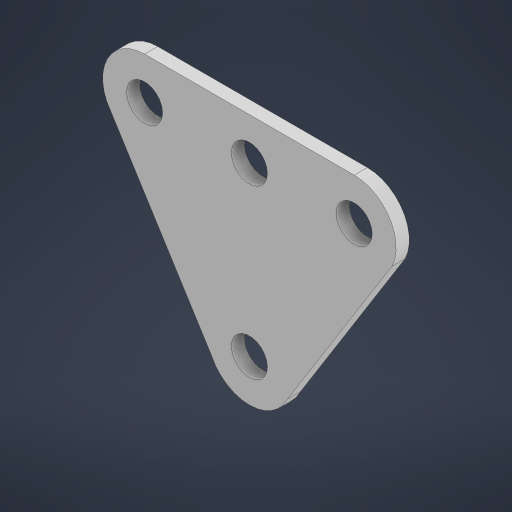
# Autodesk Inventor part: Wing poly connection
Saved by Autodesk Inventor 2023.4 (Build 274418000, 418)
## iProperties
Created: 2024-01-13
Part Number: Wing poly connection
Material: Generic
Document SubType Name: Modeling
Designer: diego
Density: 1 g/cm^3
Appearance: Default
Author: diego
Autodesk Inventor part; units mm, degrees
ref_plane "YZ Plane" through (0, 0, 0) normal (1, 0, 0) x (0, 1, 0)
ref_plane "XZ Plane" through (0, 0, 0) normal (0, 1, 0) x (-1, 0, 0)
ref_plane "XY Plane" through (0, 0, 0) normal (0, 0, 1) x (1, 0, 0)
sketch "Sketch3" plane through (0, 0, 0) normal (0, 0, 1) x (1, 0, 0)
  circle A0 centre (1.4019, 6.1779) radius 2.1844
  circle A1 centre (-11.2981, 6.1779) radius 2.1844
  circle A2 centre (-23.9981, 6.1779) radius 2.1844
  circle A3 centre (14.1019, 6.1779) radius 2.1844
  line L0 (-11.2981, 6.1779) -> (1.4019, 6.1779)
  line L1 (1.4019, 6.1779) -> (14.1019, 6.1779)
  circle A4 centre (-11.2981, 6.1779) radius 5.08
  circle A5 centre (1.4019, 6.1779) radius 5.08
  circle A6 centre (14.1019, 6.1779) radius 5.08
  line L2 (-11.2981, 11.2579) -> (1.4019, 11.2579)
  line L3 (1.4019, 11.2579) -> (14.1019, 11.2579)
  line L4 (1.4019, 6.1779) -> (1.4019, -14.1421)
  circle A7 centre (1.4019, -14.1421) radius 5.08
  circle A8 centre (1.4019, -14.1421) radius 2.1844
  line L5 (-15.8845, 3.9935) -> (-3.1845, -16.3265)
  line L6 (5.9882, -16.3265) -> (18.6882, 3.9935)
  point P0 (0, 0)
  dimension "d55" = 10.16
  dimension "d54" = 10.16
  dimension "d56" = 10.16
  dimension "d57" = 20.32
  dimension "d58" = 10.16
  dimension "d59" = 4.3688
  dimension "d60" = 4.3688
  constraints: 14 end point, 8 centre point, 6 point on circle, 5 coincident, 2 horizontal, 1 collinear, 1 point on line, 1 vertical, 1 vertical alignment, 2 other
  measures "d54" diameter of A4
  measures "d56" diameter of A6
  measures "d57" distance of L4.start L4.end
  measures "d58" diameter of A7
  measures "d59" diameter of A3
  measures "d60" diameter of A8
extrude "Extrusion7" add sketch "Sketch3" along normal blind 1.5875 contours L1 A5 L4 A0 | A0 L0 A5 L1 | A0 L4 A5 L0 | A5 L3 A6 L1 | L1 A6 L6 A7 L4 A5 | A5 L4 A7 L5 A4 L0 | L0 A4 L2 A5 | A6 L6 | A4 L5 | A7 picked at (10.0596, 5.5898) picked at (-7.2558, 5.5898)
body "Solid7"
